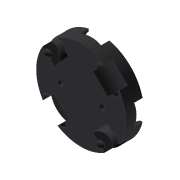
# Autodesk Inventor part: omni_wheel_core_2
Saved by Autodesk Inventor 2017 (Build 210142000, 142)
## iProperties
Created: 2018-10-27
Part Number: omni_wheel_core_2
Material: Generic
Document SubType Name: Modeling
Designer: mfans
Density: 1 g/cm^3
Appearance: Default
Author: mfans
Autodesk Inventor part; units mm, degrees
ref_plane "YZ Plane" through (0, 0, 0) normal (1, 0, 0) x (0, 1, 0)
ref_plane "XZ Plane" through (0, 0, 0) normal (0, 1, 0) x (-1, 0, 0)
ref_plane "XY Plane" through (0, 0, 0) normal (0, 0, 1) x (1, 0, 0)
sketch "Sketch1" plane through (0, 0, 0) normal (0, 1, 0) x (-1, 0, 0)
  circle A0 centre (0, 0) radius 30
  line L0 (-25, 7) -> (-18, 7)
  line L1 (-18, 7) -> (-18, -7)
  line L2 (-18, -7) -> (-25, -7)
  line L3 (-25, -7) -> (-25, 7)
  line L4 (-25, 7) -> (-18, -7) construction
  line L5 (-18, 7) -> (-25, -7) construction
  line L6 (-25, 7) -> (-25, 9.5)
  line L7 (-25, 7) -> (-22.5, 7)
  arc A1 (-22.5, 7) -> (-25, 9.5) centre (-25, 7) ccw
  line L8 (-25, -7) -> (-25, -9.5)
  line L9 (-25, -7) -> (-22.5, -7)
  arc A2 (-25, -9.5) -> (-22.5, -7) centre (-25, -7) ccw
  point P0 (-21.5, 0)
  dimension "d0" = 60
  dimension "d1" = 18
  dimension "d2" = 7
  dimension "d3" = 14
  dimension "d4" = 0
  dimension "d5" = 2.5
  dimension "d6" = 2.5
  dimension "d7" = 2.5
  dimension "d8" = 2.5
  dimension "d9" = 2.5
  dimension "d10" = 2.5
  constraints: 20 end point, 4 point on circle, 3 centre point, 2 midpoint, 2 parallel, 2 point on line, 2 vertical, 1 coincident, 1 horizontal, 1 perpendicular
  measures "d0" diameter of A0
  measures "d1" distance from line of point (0, 0) L1
  measures "d2" distance of L1.end L2.end
  measures "d3" distance of L0.end L1.end
  measures "d4" vertical distance of point (0, 0) point (-21.5, 0)
  measures "d5" distance of L0.start L6.end
  measures "d6" distance of L0.start L7.end
  measures "d7" radius of A1
  measures "d8" distance of L2.end L8.end
  measures "d9" distance of L2.end L9.end
  measures "d10" radius of A2
extrude "Extrusion1" add sketch "Sketch1" along normal mid plane 12 contours A0 | L6 A1 L0 | L0 L1 L2 L3 | L2 A2 L8
sketch "Sketch2" plane through (0, 6, 0) normal (0, 1, 0) x (1, 0, 0)
  line L0 (25, 7) -> (18, 7)
  line L1 (18, 7) -> (18, -7)
  line L2 (18, -7) -> (25, -7)
  line L3 (25, -7) -> (25, 7)
  line L4 (25, 7) -> (18, -7) construction
  line L5 (18, 7) -> (25, -7) construction
  arc A0 (25, -4.5) -> (25, -9.5) centre (25, -7) ccw
  arc A1 (25, 9.5) -> (25, 4.5) centre (25, 7) ccw
  line L6 (25, -9.5) -> (25, 9.5)
  point P0 (0, 0)
  point P1 (21.5, 0)
  dimension "d13" = 18
  dimension "d14" = 7
  dimension "d15" = 14
  dimension "d16" = 0
  dimension "d17" = 5
  dimension "d18" = 5
  constraints: 14 end point, 4 point on circle, 3 point on line, 2 centre point, 2 midpoint, 2 parallel, 1 coincident, 1 horizontal, 1 perpendicular, 1 vertical
  measures "d13" distance from line of point (0, 0) L1
  measures "d14" distance of L0.start L0.end
  measures "d15" distance of L0.end L1.end
  measures "d16" vertical distance of point (0, 0) point (21.5, 0)
  measures "d17" diameter of A0
  measures "d18" diameter of A1
revolve "Revolution1" cut sketch "Sketch2" angle 360 about axis through (25, 6, 9.5) along (0, 0, -1)
pattern_circular "Circular Pattern1" count 4 over 360 about axis through (0, -10, 0) along (0, 1, 0) of "Revolution1"
sketch "Sketch3" plane through (0, -6, 0) normal (0, -1, 0) x (1, 0, 0)
  circle A0 centre (0, 0) radius 30 projected
  line L0 (0, 0) -> (-30, 0)
  line L1 (0, 0) -> (-17.6777, 17.6777)
  line L2 (-7.7782, 17.6777) -> (-17.6777, 7.7782)
  line L3 (-27.5772, 17.6777) -> (-17.6777, 27.5772)
  line L4 (-17.6777, 27.5772) -> (-17.6777, 7.7782) construction
  line L5 (-7.7782, 17.6777) -> (-27.5772, 17.6777) construction
  arc A1 (-14.4957, 20.8597) -> (-10.9602, 24.3952) centre (-12.7279, 22.6274) ccw
  arc A2 (-24.3952, 10.9602) -> (-20.8597, 14.4957) centre (-22.6274, 12.7279) ccw
  line L6 (-10.9602, 24.3952) -> (-24.3952, 10.9602)
  line L7 (-17.6777, 27.5772) -> (-14.4957, 24.3952)
  line L8 (-12.7279, 22.6274) -> (-7.7782, 17.6777)
  line L9 (-17.6777, 7.7782) -> (-22.6274, 12.7279)
  line L10 (-24.3952, 14.4957) -> (-27.5772, 17.6777)
  dimension "d23" = 25
  dimension "d24" = 45
  dimension "d25" = 14
  dimension "d26" = 90
  dimension "d27" = 14
  dimension "d28" = 5
  dimension "d29" = 5
  constraints: 22 end point, 5 parallel, 4 point on circle, 4 point on line, 2 centre point, 2 midpoint, 2 perpendicular, 1 horizontal, 1 horizontal alignment, 1 other
  measures "d23" distance of L0.start L1.end
  measures "d24" angle of L0 L1
  measures "d25" distance of L2.end L3.start
  measures "d26" angle of L1 L2
  measures "d27" distance of L2.start L2.end
  measures "d28" diameter of A1
  measures "d29" diameter of A2
revolve "Revolution2" cut sketch "Sketch3" angle 360 about axis through (-10.9602, -6, 24.3952) along (-0.7071, 0, -0.7071) contours L2 L9 A2 L6 L1 | L1 L6 A1 L8 L2 | L6 L8 A1 | A2 L9 L6 | L8 L6 A1 | A2 L6 L9
pattern_circular "Circular Pattern2" count 4 over 360 about axis through (0, -10, 0) along (0, 1, 0) of "Revolution2"
sketch "Sketch4" plane through (0, 6, 0) normal (0, 1, 0) x (1, 0, 0)
  point P0 (0, 0)
  point P1 (-14, 0)
  point P2 (14, 0)
  dimension "d34" = 14
  dimension "d35" = 14
  measures "d34" distance of point (14, 0) point (0, 0)
  measures "d35" distance of point (-14, 0) point (0, 0)
hole "Hole1" at (-14, 6, 0) at (14, 6, 0) direction (0, -1, 0) diameter 4 end through all
body "Solid1"
